Autodesk Inventor part; units mm, degrees
(part 2 of 2)
  line L67 (-3.9525, 47.2916) -> (-6.704, 47.2916)
  line L68 (-3.5575, 47.6451) -> (-3.8818, 47.3209)
  arc A18 (-19.8782, 57.6416) -> (-19.9782, 57.5416) centre (-19.8782, 57.5416) ccw
  line L69 (-14.9908, 57.6416) -> (-10.7025, 57.6416)
  line L70 (0, 60) -> (-10, 60)
  line L71 (0, 60) -> (-21.0398, 60)
  line L72 (-21.0398, 60) -> (-21.0398, 45.6746)
  line L73 (-21.0398, 45.6746) -> (0, 45.6746)
  line L74 (0, 45.6746) -> (0, 60)
  point P0 (0, 30)
  point P1 (0, 30)
  constraints: 150 end point, 34 point on circle, 19 centre point, 4 symmetric about line, 2 parallel, 1 horizontal, 1 perpendicular, 74 other
extrude "Выдавливание4" [suppressed]
